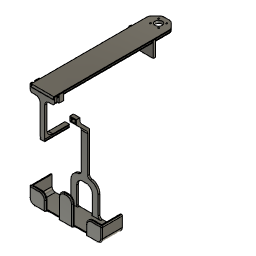
HeliumAntennaMount (Autodesk Fusion 360 design; units mm, degrees)
Autodesk Fusion 360 part; units mm, degrees
note: some values were not read from the file. Set by a fixed rule: which sketch regions a step uses.
sketch "Sketch1" plane through (0, 0, 0) normal (0, 0, 1) x (1, 0, 0)
  line L0 (0, -99.1) -> (0, 467.9) construction
  line L1 (-25, 0) -> (25, 0)
  line L2 (25, 0) -> (25, 275)
  line L3 (25, 275) -> (-25, 275)
  line L4 (-25, 275) -> (-25, 0)
  line L5 (-101.9, 257) -> (109.8, 257) construction
  circle A0 centre (0, 257) radius 8.12
  line L6 (-140.1, 0) -> (138.6, 0) construction
  dimension "d1" = 50
  dimension "d2" = 275
  dimension "d3" = 18
  dimension "d4" = 16.24
  constraint vertical L0
  constraint horizontal L1
  constraint vertical L2
  constraint horizontal L3
  constraint vertical L4
  constraint symmetric L0 L2 L4
  constraint perpendicular L2 L5
  constraint coincident L0 A0.centre
  constraint coincident L5 A0.centre
  constraint horizontal L6
  constraint collinear L1 L6
  measures "d1" distance of L1.start L1.end
  measures "d2" distance of L1.start L3.end
  measures "d3" distance of L3 L5
  measures "d4" diameter of A0
extrude "Extrude1" add sketch "Sketch1" along normal blind 6 makes body 1
sketch "Sketch2" plane through (0, 0, 0) normal (0, 0, -1) x (1, 0, 0)
  circle A0 centre (0, -257) radius 8.12
  line L0 (-25, 0) -> (-25, -275)
  line L1 (-25, -275) -> (25, -275)
  line L2 (25, -275) -> (25, 0)
  line L3 (25, 0) -> (-25, 0)
sketch "Sketch3" plane through (0, 0, 6) normal (0, 0, 1) x (-1, 0, 0)
  circle A0 centre (0, -257) radius 8.12
  line L0 (25, -275) -> (25, 0)
  line L1 (25, 0) -> (-25, 0)
  line L2 (-25, 0) -> (-25, -275)
  line L3 (-25, -275) -> (25, -275)
  line L4 (-9, -266) -> (9, -266) construction
  line L5 (9, -266) -> (9, -248) construction
  line L6 (9, -248) -> (-9, -248) construction
  line L7 (-9, -248) -> (-9, -266) construction
  line L8 (-9, -266) -> (9, -248) construction
  line L9 (9, -266) -> (-9, -248) construction
  circle A1 centre (9, -266) radius 1.625
  circle A2 centre (9, -248) radius 1.625
  circle A3 centre (-9, -248) radius 1.625
  circle A4 centre (-9, -266) radius 1.625
  point P0 (0, -257)
  dimension "d7" = 18
  dimension "d8" = 18
  dimension "d9" = 3.25
  dimension "d10" = 3.25
  dimension "d11" = 3.25
  dimension "d12" = 3.25
  constraint horizontal L4
  constraint perpendicular L4 L5
  constraint parallel L4 L6
  constraint parallel L5 L7
  constraint coincident L8 P0
  constraint coincident L9 P0
  constraint coincident P0 A0.centre
  constraint coincident L4.end L5.start
  constraint coincident L5.end L6.start
  constraint coincident L6.end L7.start
  constraint coincident L4.start L7.end
  measures "d7" distance of L5.end L6.end
  measures "d8" distance of L4.end L5.end
  measures "d9" diameter of A1
  measures "d10" diameter of A2
  measures "d11" diameter of A3
  measures "d12" diameter of A4
extrude "Extrude2" cut sketch "Sketch3" against normal up to surface (6 mm away) contours A1 | A2 | A3 | A4 bodies 1
chamfer "Chamfer1" distance 15 angle 45 1 edges at (-25, 275, 3) on bodies 1
chamfer "Chamfer2" distance 15 angle 45 1 edges at (25, 275, 3) on bodies 1
fillet "Fillet1" radius 10 4 edges at (10, 275, 3) (-10, 275, 3) (-25, 260, 3) (25, 260, 3) on bodies 1
sketch "Sketch6" plane through (0, 0, 0) normal (0, -1, 0) x (1, 0, 0)
  line L0 (-25, 0) -> (25, 0)
  line L1 (25, 0) -> (25, 6)
  line L2 (25, 6) -> (-25, 6)
  line L3 (-25, 6) -> (-25, 0)
  line L4 (-26.4781, 3) -> (26.4, 3) construction
  line L5 (-26.4, 4.5) -> (26.8, 4.5) construction
  line L6 (-26.4, 1.5) -> (26.8, 1.5) construction
  line L7 (-23.5, 6.3) -> (-23.5, 0.2) construction
  line L8 (-25, 1.5) -> (-23.5, 3)
  line L9 (-25, 4.5) -> (-23.5, 3)
  line L10 (0, 7.5) -> (0, -2.9) construction
  line L11 (25, 4.5) -> (23.5, 3)
  line L12 (25, 1.5) -> (23.5, 3)
  dimension "d28" = 1.5
  dimension "d29" = 1.5
  constraint perpendicular L1 L4
  constraint perpendicular L1 L5
  constraint symmetric L4 L5.start L6.start
  constraint symmetric L4 L5.end L6.end
  constraint perpendicular L6 L7
  constraint coincident L6 L8.start
  constraint coincident L3 L8.start
  constraint coincident L4 L8.end
  constraint coincident L7 L8.end
  constraint coincident L5 L9.start
  constraint coincident L3 L9.start
  constraint perpendicular L0 L10
  constraint symmetric L8.start L10 L12.start
  constraint symmetric L8.end L10 L11.end
  constraint symmetric L9.start L10 L11.start
  measures "d28" distance of L4 L5
  measures "d29" distance of L3 L7
extrude "Extrude6" cut sketch "Sketch6" against normal up to surface (275 mm away) contours L3 L8 L9 | L1 L11 L12 bodies 1
copy_body "Body->Comp1" bodies 1 removing the originals makes body 2 in component "Bodey"
sketch "Sketch1 (2)" plane through (0, 0, 0) normal (0, 1, 0) x (1, 0, 0) in component "Leg 1"
  line L0 (-25, -4.5) -> (-23.5, -3)
  line L1 (-23.5, -3) -> (-25, -1.5)
  line L2 (-25, -1.5) -> (-25, 0)
  line L3 (-25, 0) -> (25, 0)
  line L4 (25, 0) -> (25, -1.5)
  line L5 (25, -1.5) -> (23.5, -3)
  line L6 (23.5, -3) -> (25, -4.5)
  line L7 (25, -4.5) -> (25, -6)
  line L8 (-25, -6) -> (-25, -4.5)
  line L9 (-25.15, -6) -> (-25.15, -4.4379)
  line L10 (-25.15, -4.4379) -> (-23.7121, -3)
  line L11 (-23.7121, -3) -> (-25.15, -1.5621)
  line L12 (-25.15, -1.5621) -> (-25.15, 0.15)
  line L13 (-25.15, 0.15) -> (25.15, 0.15)
  line L14 (25.15, 0.15) -> (25.15, -1.5621)
  line L15 (25.15, -1.5621) -> (23.7121, -3)
  line L16 (23.7121, -3) -> (25.15, -4.4379)
  line L17 (25.15, -4.4379) -> (25.15, -6)
  line L18 (-25.15, -6) -> (-27.15, -6)
  line L19 (-27.15, -6) -> (-27.15, 10.15)
  line L20 (-27.15, 10.15) -> (0, 10.15)
  line L21 (0, 15.35) -> (0, 0.25) construction
  line L22 (25.15, -6) -> (27.15, -6)
  line L23 (27.15, -6) -> (27.15, 10.15)
  line L24 (27.15, 10.15) -> (0, 10.15)
  line L25 (-27.8377, 0.15) -> (28.2, 0.15) construction
  line L26 (-5, 10.15) -> (-5, 90.15)
  line L27 (5, 10.15) -> (5, 90.15)
  line L28 (-5, 90.15) -> (5, 90.15)
  dimension "d32" = -0.15
  dimension "d33" = 2
  dimension "d36" = 10
  dimension "d43" = 80
  dimension "d44" = 5
  constraint perpendicular L9 L18
  constraint perpendicular L18 L19
  constraint perpendicular L19 L20
  constraint perpendicular L3 L21
  constraint symmetric L9.start L21 L17.end
  constraint symmetric L18.end L21 L22.end
  constraint symmetric L19.end L21 L23.end
  constraint symmetric L20.end L21 L24.end
  constraint parallel L3 L25
  constraint coincident L20 L26.start
  constraint perpendicular L20 L26
  constraint symmetric L21 L26.start L27.start
  constraint symmetric L21 L26.end L27.end
  measures "d33" distance of L9.start L18.end
  measures "d36" distance of L20 L25
  measures "d43" distance of L26.start L26.end
  measures "d44" distance of L21 L26
extrude "Extrude5" add sketch "Sketch1 (2)" along normal blind 5 separate body makes body 3 in component "Leg 1"
extrude "Extrude3" add sketch "Sketch1 (2)" along normal blind 10 separate body contours L9 L10 L11 L12 L13 L14 L15 L16 L17 L18 L19 L20 L22 L23 L24 makes body 4 in component "Leg 1"
extrude "Extrude1'" add sketch "Sketch1 (2)" along normal blind 5 separate body contours L9 L10 L11 L12 L13 L14 L15 L16 L17 L18 L19 L20 L22 L23 L24 makes body 5 in component "Leg 1"
move_body "Move1" bodies 5 to x (1, 0, 0) y (0, 1, 0) z (0, 0, 1) at (0, 218.5, 0) in component "Leg 1"
sketch "Sketch2 (2)" plane through (0, 0, -10.15) normal (0, 0, -1) x (1, 0, 0) in component "Leg 1"
  line L0 (27.15, -218.5) -> (-27.15, -218.5)
  line L1 (-27.15, -218.5) -> (-27.15, -223.5)
  line L2 (-27.15, -223.5) -> (27.15, -223.5)
  line L3 (27.15, -223.5) -> (27.15, -218.5)
move_body "Move2" bodies 4 to x (1, 0, 0) y (0, 1, 0) z (0, 0, 1) at (0, 10, 0) in component "Leg 1"
extrude "Extrude4" add sketch "Sketch2 (2)" along normal blind 18.5 bodies 5 in component "Leg 1"
sketch "Sketch3 (2)" plane through (0, 5, 0) normal (0, 1, 0) x (-1, 0, 0) in component "Leg 1"
  line L0 (25.15, 6) -> (25.15, 4.4379)
  line L1 (25.15, 4.4379) -> (23.7121, 3)
  line L2 (23.7121, 3) -> (25.15, 1.5621)
  line L3 (25.15, 1.5621) -> (25.15, -0.15)
  line L4 (25.15, -0.15) -> (-25.15, -0.15)
  line L5 (-25.15, -0.15) -> (-25.15, 1.5621)
  line L6 (-25.15, 1.5621) -> (-23.7121, 3)
  line L7 (-23.7121, 3) -> (-25.15, 4.4379)
  line L8 (-25.15, 4.4379) -> (-25.15, 6)
  line L9 (-25.15, 6) -> (-27.15, 6)
  line L10 (-27.15, 6) -> (-27.15, -10.15)
  line L11 (-27.15, -10.15) -> (-5, -10.15)
  line L12 (-5, -10.15) -> (-5, -90.15)
  line L13 (-5, -90.15) -> (5, -90.15)
  line L14 (5, -90.15) -> (5, -10.15)
  line L15 (5, -10.15) -> (27.15, -10.15)
  line L16 (27.15, -10.15) -> (27.15, 6)
  line L17 (27.15, 6) -> (25.15, 6)
  line L18 (0, -57.1) -> (0, 9.3) construction
  line L19 (-5, -90.15) -> (5, -90.15)
  line L20 (5, -90.15) -> (5, -84.15)
  line L21 (5, -84.15) -> (-5, -84.15)
  line L22 (-5, -84.15) -> (-5, -90.15)
  dimension "d47" = 6
  constraint perpendicular L4 L18
  constraint horizontal L19
  constraint vertical L20
  constraint horizontal L21
  constraint vertical L22
  constraint coincident L12.end L13.start
  measures "d47" distance of L12.end L21.end
extrude "Extrude6'" add sketch "Sketch3 (2)" along normal blind 50 contours L12 L13 L14 L19 L20 L21 L22 bodies 3 in component "Leg 1"
sketch "Sketch4" plane through (0, 55, 0) normal (0, 1, 0) x (-1, 0, 0) in component "Leg 1"
  line L0 (-5, -84.15) -> (-5, -90.15)
  line L1 (-5, -90.15) -> (5, -90.15)
  line L2 (5, -90.15) -> (5, -84.15)
  line L3 (5, -84.15) -> (-5, -84.15)
  line L4 (-5, -87.15) -> (5, -87.15) construction
  line L5 (-5, -85.65) -> (5, -85.65) construction
  line L6 (-5, -88.65) -> (5, -88.65) construction
  line L7 (-3.5, -90.8) -> (-3.5, -84.15) construction
  line L8 (-3.5, -87.15) -> (-5, -88.65)
  line L9 (-3.5, -87.15) -> (-5, -85.65)
  line L10 (0, -91.3) -> (0, -83.7) construction
  line L11 (3.5, -87.15) -> (5, -85.65)
  line L12 (3.5, -87.15) -> (5, -88.65)
  dimension "d50" = 1.5
  dimension "d51" = 1.5
  constraint midpoint L0 L4.start
  constraint midpoint L2 L4.end
  constraint coincident L0 L5.start
  constraint coincident L2 L5.end
  constraint perpendicular L2 L5
  constraint symmetric L4 L5.start L6.start
  constraint symmetric L4 L5.end L6.end
  constraint coincident L3 L7.end
  constraint perpendicular L3 L7
  constraint coincident L4 L8.start
  constraint coincident L7 L8.start
  constraint perpendicular L3 L10
  constraint symmetric L5.start L10 L5.end
  constraint symmetric L6.start L10 L6.end
  constraint symmetric L8.start L10 L11.start
  measures "d50" distance of L4 L5
  measures "d51" distance of L0 L7
extrude "Extrude7" cut sketch "Sketch4" against normal up to surface (55 mm away) contours L0 L8 L9 | L2 L11 L12 bodies 3 in component "Leg 1"
fillet "Fillet1'" radius 13.25 1 edges at (0, 5, -84.15) on bodies 3 in component "Leg 1"
fillet "Fillet2" radius 10 1 edges at (-5, 2.5, -10.15) on bodies 3 in component "Leg 1"
fillet "Fillet3" radius 10 1 edges at (5, 2.5, -10.15) on bodies 3 in component "Leg 1"
fillet "Fillet4" radius 5 1 edges at (27.15, 2.5, -10.15) on bodies 3 in component "Leg 1"
fillet "Fillet5" radius 5 1 edges at (-27.15, 2.5, -10.15) on bodies 3 in component "Leg 1"
sketch "Sketch1 (3)" plane through (0, 55, 0) normal (0, 1, 0) x (-1, 0, 0) in component "Holster"
  line L0 (-3.5, -87.15) -> (-5, -88.65)
  line L1 (-5, -88.65) -> (-5, -90.15)
  line L2 (-5, -90.15) -> (5, -90.15)
  line L3 (5, -90.15) -> (5, -88.65)
  line L4 (5, -88.65) -> (3.5, -87.15)
  line L5 (3.5, -87.15) -> (5, -85.65)
  line L6 (5, -85.65) -> (5, -84.15)
  line L7 (5, -84.15) -> (-5, -84.15)
  line L8 (-5, -84.15) -> (-5, -85.65)
  line L9 (-5, -85.65) -> (-3.5, -87.15)
  line L10 (-5.15, -85.7121) -> (-3.7121, -87.15)
  line L11 (-3.7121, -87.15) -> (-5.15, -88.5879)
  line L12 (-5.15, -88.5879) -> (-5.15, -90.3)
  line L13 (-5.15, -90.3) -> (5.15, -90.3)
  line L14 (5.15, -90.3) -> (5.15, -88.5879)
  line L15 (5.15, -88.5879) -> (3.7121, -87.15)
  line L16 (3.7121, -87.15) -> (5.15, -85.7121)
  line L17 (5.15, -85.7121) -> (5.15, -84)
  line L18 (5.15, -84) -> (-5.15, -84)
  line L19 (-5.15, -84) -> (-5.15, -85.7121)
  line L20 (-7.15, -82) -> (7.15, -82)
  line L21 (7.15, -82) -> (7.15, -92.3)
  line L22 (7.15, -92.3) -> (-7.15, -92.3)
  line L23 (-7.15, -92.3) -> (-7.15, -82)
  dimension "d59" = 0.15
  dimension "d60" = 2
  dimension "d61" = 2
  dimension "d62" = 2
  dimension "d63" = 2
  constraint horizontal L20
  constraint vertical L21
  constraint horizontal L22
  constraint vertical L23
  measures "d60" distance of L18 L20
  measures "d61" distance of L13 L22
  measures "d62" distance of L12 L23
  measures "d63" distance of L14 L21
extrude "Extrude1''" add sketch "Sketch1 (3)" along normal blind 8 separate body contours L20 L21 L22 L23 makes body 6 in component "Holster"
ref_plane "WorkPlane1" through (7.15, 59, -87.15) normal (1, 0, 0) x (0, 0, -1)
sketch "Sketch7" plane through (7.15, 59, -87.15) normal (1, 0, 0) x (0, 1, 0)
  line L0 (-4, -5.15) -> (17.2132, -26.3632)
  line L1 (-4, -5.15) -> (26, -5.15) construction
  line L2 (17.2132, -26.3632) -> (25.2132, -26.3632)
  line L3 (25.2132, -26.3632) -> (4, -5.15)
  line L4 (4, -5.15) -> (-4, -5.15)
  point P0 (-4, -5.15)
  point P1 (4, -5.15)
  dimension "d67" = 30
  dimension "d68" = 45
  dimension "d69" = 8
  constraint horizontal L1
  constraint coincident P0 L0.start
  constraint horizontal L2
  constraint coincident P1 L3.end
  measures "d67" distance of P0 L0.end
  measures "d68" angle of L0 L1
  measures "d69" distance of L0.end L2.end
extrude "Extrude2'" add sketch "Sketch7" against normal blind 14.3 bodies 6 in component "Holster"
sketch "Sketch8" plane through (-7.15, 0, 0) normal (-1, 0, 0) x (0, -1, 0)
  line L0 (-55, -92.3) -> (-55, -82)
  line L1 (-55, -82) -> (-63, -82)
  line L2 (-63, -82) -> (-63, -92.3)
  line L3 (-63, -92.3) -> (-84.2132, -113.5132)
  line L4 (-84.2132, -113.5132) -> (-76.2132, -113.5132)
  line L5 (-76.2132, -113.5132) -> (-55, -92.3)
  line L6 (-84.2132, -113.5132) -> (-84.2132, -273.5132)
  line L7 (-84.2132, -273.5132) -> (-80.2132, -273.5132)
  line L8 (-80.2132, -273.5132) -> (-80.2132, -113.5132)
  dimension "d73" = 160
  dimension "d74" = 4
  constraint coincident L3.end L4.start
  constraint perpendicular L4 L6
  constraint perpendicular L6 L7
  constraint midpoint L4 L8.end
  measures "d73" distance of L3.end L6.end
  measures "d74" distance of L6.end L7.end
extrude "Extrude3'" add sketch "Sketch8" against normal up to surface (14.3 mm away) contours L4 L6 L7 L8 bodies 6 in component "Holster"
fillet "Fillet1''" radius 13 1 edges at (0, 63, -92.3) on bodies 6 in component "Holster"
fillet "Fillet2'" radius 9.5 1 edges at (0, 80.2132, -113.5132) on bodies 6 in component "Holster"
sketch "Sketch18" plane through (0, 0, -273.5132) normal (0, 0, -1) x (1, 0, 0)
  line L0 (7.15, -84.2132) -> (7.15, -80.2132)
  line L1 (7.15, -80.2132) -> (-7.15, -80.2132)
  line L2 (-7.15, -80.2132) -> (-7.15, -84.2132)
  line L3 (-7.15, -84.2132) -> (7.15, -84.2132)
  line L4 (0, -80.2132) -> (0, -85.7)
  line L5 (-76, -42.2132) -> (76, -42.2132)
  line L6 (76, -42.2132) -> (76, -80.2132)
  line L7 (76, -80.2132) -> (-76, -80.2132)
  line L8 (-76, -80.2132) -> (-76, -42.2132)
  dimension "d134" = 152
  dimension "d135" = 38
  constraint midpoint L1 L4.start
  constraint perpendicular L3 L4
  constraint horizontal L5
  constraint vertical L6
  constraint horizontal L7
  constraint vertical L8
  constraint midpoint L4.start L7
  measures "d134" distance of L5.start L5.end
  measures "d135" distance of L5.start L7.end
extrude "Extrude7'" add sketch "Sketch18" along normal blind 4 separate body contours L1 L5 L6 L7 L8 makes body 7
sketch "Sketch19" plane through (0, 80.2132, 0) normal (0, 1, 0) x (-1, 0, 0)
  line L0 (76, -273.5132) -> (-76, -273.5132)
  line L1 (-76, -273.5132) -> (-76, -277.5132)
  line L2 (-76, -277.5132) -> (76, -277.5132)
  line L3 (76, -277.5132) -> (76, -273.5132)
extrude "Extrude8" add sketch "Sketch19" along normal up to surface (4 mm away) bodies 7
sketch "Sketch20" plane through (-76, 0, 0) normal (-1, 0, 0) x (0, -1, 0)
  line L0 (-42.2132, -273.5132) -> (-84.2132, -273.5132)
  line L1 (-84.2132, -273.5132) -> (-84.2132, -277.5132)
  line L2 (-84.2132, -277.5132) -> (-42.2132, -277.5132)
  line L3 (-42.2132, -277.5132) -> (-42.2132, -273.5132)
  line L4 (-42.2132, -277.5132) -> (-103.2132, -277.5132)
  line L5 (-103.2132, -277.5132) -> (-103.2132, -242.5132)
  line L6 (-103.2132, -242.5132) -> (-42.2132, -242.5132)
  line L7 (-42.2132, -242.5132) -> (-42.2132, -277.5132)
  dimension "d140" = 35
  constraint horizontal L4
  constraint vertical L5
  constraint horizontal L6
  constraint vertical L7
  constraint coincident L2.end L3.start
  measures "d140" distance of L2.end L6.end
extrude "Extrude9" add sketch "Sketch20" along normal blind 4 separate body contours L0 L1 L4 L5 L6 L7 makes body 8
sketch "Sketch21" plane through (0, 0, -273.5132) normal (0, 0, -1) x (1, 0, 0)
  line L0 (-76, -84.2132) -> (-76, -42.2132)
  line L1 (-76, -42.2132) -> (-80, -42.2132)
  line L2 (-80, -42.2132) -> (-80, -84.2132)
  line L3 (-80, -84.2132) -> (-76, -84.2132)
extrude "Extrude10" add sketch "Sketch21" along normal up to surface (4 mm away) bodies 7 8
ref_plane "WorkPlane3" through (76, 72.7132, -260.0132) normal (1, 0, 0) x (0, 1, 0)
sketch "Sketch22" plane through (76, 53.7132, -258.0132) normal (1, 0, 0) x (0, 1, 0)
  line L0 (49.5, -19.5) -> (-11.5, -19.5)
  line L1 (-11.5, -19.5) -> (-11.5, 15.5)
  line L2 (-11.5, 15.5) -> (49.5, 15.5)
  line L3 (49.5, 15.5) -> (49.5, -19.5)
extrude "Extrude11" add sketch "Sketch22" along normal blind 4 bodies 7
sketch "Sketch23" plane through (0, 42.2132, 0) normal (0, -1, 0) x (1, 0, 0)
  line L0 (-80, -242.5132) -> (-80, -277.5132)
  line L1 (-80, -277.5132) -> (80, -277.5132)
  line L2 (80, -277.5132) -> (80, -242.5132)
  line L3 (80, -242.5132) -> (76, -242.5132)
  line L4 (76, -242.5132) -> (76, -273.5132)
  line L5 (76, -273.5132) -> (-76, -273.5132)
  line L6 (-76, -273.5132) -> (-76, -242.5132)
  line L7 (-76, -242.5132) -> (-80, -242.5132)
  line L8 (-80, -242.5132) -> (-45, -242.5132)
  line L9 (-45, -242.5132) -> (-45, -277.5132)
  line L10 (-45, -277.5132) -> (-80, -277.5132)
  line L11 (-80, -277.5132) -> (-80, -242.5132)
  line L12 (80, -242.5132) -> (45, -242.5132)
  line L13 (45, -242.5132) -> (45, -277.5132)
  line L14 (45, -277.5132) -> (80, -277.5132)
  line L15 (80, -277.5132) -> (80, -242.5132)
  dimension "d148" = 35
  dimension "d149" = 35
  constraint horizontal L8
  constraint vertical L9
  constraint horizontal L10
  constraint vertical L11
  constraint coincident L1 L9.end
  constraint coincident L0.start L7.end
  constraint horizontal L12
  constraint vertical L13
  constraint horizontal L14
  constraint vertical L15
  constraint coincident L1 L13.end
  constraint coincident L2.end L3.start
  measures "d148" distance of L0.start L8.end
  measures "d149" distance of L2.end L12.end
extrude "Extrude12" add sketch "Sketch23" along normal blind 4 contours L0 L1 L5 L6 L7 L8 L9 L10 L11 | L5 L6 L8 L9 | L1 L2 L3 L4 L5 L12 L13 L14 L15 | L4 L5 L12 L13 bodies 7
sketch "Sketch24" plane through (0, 42.2132, 0) normal (0, -1, 0) x (1, 0, 0)
  line L0 (-45, -273.5132) -> (-45, -277.5132)
  line L1 (-45, -277.5132) -> (45, -277.5132)
  line L2 (45, -277.5132) -> (45, -273.5132)
  line L3 (45, -273.5132) -> (-45, -273.5132)
  line L4 (7.15, -273.5132) -> (7.15, -121.2592)
  line L5 (-26.7, -248.5132) -> (32.5, -248.5132) construction
  line L6 (-15.1892, -277.5132) -> (15.1892, -277.5132)
  line L7 (15.1892, -277.5132) -> (15.1892, -219.5132)
  line L8 (15.1892, -219.5132) -> (-15.1892, -219.5132)
  line L9 (-15.1892, -219.5132) -> (-15.1892, -277.5132)
  line L10 (-15.1892, -277.5132) -> (15.1892, -219.5132) construction
  line L11 (15.1892, -277.5132) -> (-15.1892, -219.5132) construction
  point P0 (0, -248.5132)
  dimension "d152" = 25
  constraint perpendicular L4 L5
  constraint horizontal L6
  constraint perpendicular L6 L7
  constraint parallel L6 L8
  constraint parallel L7 L9
  constraint coincident L1 L6.start
  constraint coincident L10 P0
  constraint coincident L11 P0
  constraint coincident L5 P0
  measures "d152" distance of L3 L5.start
extrude "Extrude13" add sketch "Sketch24" along normal blind 4 contours L3 L4 L8 L9 | L1 L3 L6 L7 L9 | L3 L4 L7 L8 bodies 7
fillet "Fillet2''" radius 10.9 2 edges at (80, 70.7132, -277.5132) (-80, 70.7132, -277.5132) on bodies 7
fillet "Fillet3'" radius 7.45 2 edges at (-76, 63.2132, -273.5132) (76, 63.2132, -273.5132) on bodies 7
sketch "Sketch25" plane through (0, 0, -273.5132) normal (0, 0, -1) x (1, 0, 0)
  line L0 (7.15, -84.2132) -> (7.15, -80.2132)
  line L1 (7.15, -80.2132) -> (-7.15, -80.2132)
  line L2 (-7.15, -80.2132) -> (-7.15, -84.2132)
  line L3 (-7.15, -84.2132) -> (7.15, -84.2132)
extrude "Extrude15" add sketch "Sketch25" along normal up to surface (4 mm away) bodies 6 in component "Holster"
copy_body "CutPasteBodies1" bodies 7 removing the originals makes body 9 in component "Holster"
combine "Combine1" operation add target body 6 tool bodies 9 in component "Holster"
fillet "Fillet15" radius 5.75 2 edges at (7.15, 82.2132, -273.5132) (-7.15, 82.2132, -273.5132) on bodies 6 in component "Holster"
fillet "Fillet16" radius 12.75 4 edges at (-45, 40.2132, -242.5132) (45, 40.2132, -242.5132) (-15.1892, 40.2132, -219.5132) (15.1892, 40.2132, -219.5132) on bodies 6 in component "Holster"
fillet "Fillet17" radius 2 13 edges at (-45, 38.2132, -266.3882) (-48.7344, 38.2132, -246.2476) (-68.875, 38.2132, -242.5132) (-80, 70.7132, -242.5132) (15.1892, 38.2132, -254.8882) (11.4548, 38.2132, -223.2476) (0, 38.2132, -219.5132) (-11.4548, 38.2132, -223.2476) (-15.1892, 38.2132, -254.8882) (68.875, 38.2132, -242.5132) (48.7344, 38.2132, -246.2476) (45, 38.2132, -266.3882) (80, 70.7132, -242.5132) on bodies 6 in component "Holster"
fillet "Fillet18" radius 3.05 4 edges at (-45, 42.2132, -275.5132) (15.1892, 42.2132, -275.5132) (45, 42.2132, -275.5132) (-15.1892, 42.2132, -275.5132) on bodies 6 in component "Holster"
fillet "Fillet19" radius 2 1 edges at (0, 80.2132, -273.5132) on bodies 6 in component "Holster"
ref_plane "WorkPlane4" through (0, 84.2132, -195.5132) normal (0, 1, 0) x (0, 0, 1)
sketch "Sketch26" plane through (0, 84.2132, -195.5132) normal (0, 1, 0) x (1, 0, 0)
  arc A0 (2.4392, 24) -> (15.1892, 36.75) centre (2.4392, 36.75) ccw
  line L0 (15.1892, 36.75) -> (15.1892, 78)
  line L1 (15.1892, 78) -> (-15.1892, 78)
  line L2 (-15.1892, 78) -> (-15.1892, 36.75)
  arc A1 (-15.1892, 36.75) -> (-2.4392, 24) centre (-2.4392, 36.75) ccw
  line L3 (-2.4392, 24) -> (2.4392, 24)
  line L4 (12.9, 78) -> (-12.9, 78)
  line L5 (-12.9, 78) -> (-68.55, 78)
  line L6 (-68.55, 78) -> (-45, 78)
  line L7 (-45.0437, 78) -> (-45, 78)
  line L8 (-42.0604, 78) -> (-45.0437, 78)
  line L9 (-42.0604, 78) -> (-18.1289, 78)
  line L10 (-18.1289, 78) -> (-15.1455, 78)
  line L11 (-15.1892, 78) -> (-15.1455, 78)
  line L12 (-15.1892, 78) -> (15.1892, 78)
  line L13 (15.1455, 78) -> (15.1892, 78)
  line L14 (18.1289, 78) -> (15.1455, 78)
  line L15 (18.1289, 78) -> (42.0604, 78)
  line L16 (42.0604, 78) -> (45.0437, 78)
  line L17 (45, 78) -> (45.0437, 78)
  line L18 (45, 78) -> (68.55, 78)
  line L19 (68.55, 78) -> (12.9, 78)
  line L20 (30, 78) -> (-30, 78)
  line L21 (-30, 78) -> (-30, 11.9)
  line L22 (-30, 11.9) -> (30, 11.9)
  line L23 (30, 11.9) -> (30, 78)
  line L24 (0, 111.7) -> (0, 6.8) construction
  line L25 (-2.4392, 21.7283) -> (2.4392, 21.7283)
  arc A2 (2.4392, 21.7283) -> (17.4609, 36.75) centre (2.4392, 36.75) ccw
  line L26 (17.4609, 36.75) -> (17.4609, 80.2717)
  line L27 (17.4609, 80.2717) -> (-17.4609, 80.2717)
  line L28 (-17.4609, 80.2717) -> (-17.4609, 36.75)
  arc A3 (-17.4609, 36.75) -> (-2.4392, 21.7283) centre (-2.4392, 36.75) ccw
  dimension "d166" = 60
  dimension "d167" = 2.2717
  constraint horizontal L20
  constraint vertical L21
  constraint horizontal L22
  constraint vertical L23
  constraint coincident L15 L20.start
  constraint perpendicular L22 L24
  constraint symmetric L21 L23 L24
  measures "d166" distance of L20.start L20.end
extrude "Extrude16" add sketch "Sketch26" against normal blind 4 contours L5 L9 L10 L14 L15 L19 L20 L21 L22 L23 L25 A2 L26 L28 A3 bodies 6 in component "Holster"
sketch "Sketch27" plane through (0, 84.2132, 0) normal (0, 1, 0) x (-1, 0, 0)
  line L0 (-30, -273.5132) -> (-68.55, -273.5132)
  arc A0 (-76, -266.0632) -> (-68.55, -273.5132) centre (-68.55, -266.0632) ccw
  line L1 (-76, -266.0632) -> (-76, -275.0512)
  arc A1 (-76, -275.0512) -> (-69.1, -277.5132) centre (-69.1, -266.6132) ccw
  line L2 (-69.1, -277.5132) -> (69.1, -277.5132)
  arc A2 (69.1, -277.5132) -> (76, -275.0512) centre (69.1, -266.6132) ccw
  line L3 (76, -275.0512) -> (76, -266.0632)
  arc A3 (68.55, -273.5132) -> (76, -266.0632) centre (68.55, -266.0632) ccw
  line L4 (68.55, -273.5132) -> (30, -273.5132)
  line L5 (30, -273.5132) -> (30, -207.4132)
  line L6 (30, -207.4132) -> (7.15, -207.4132)
  line L7 (7.15, -207.4132) -> (7.15, -113.5132)
  line L8 (7.15, -113.5132) -> (-7.15, -113.5132)
  line L9 (-7.15, -113.5132) -> (-7.15, -207.4132)
  line L10 (-7.15, -207.4132) -> (-30, -207.4132)
  line L11 (-30, -207.4132) -> (-30, -273.5132)
  line L12 (-17.4609, -273.5132) -> (-17.4609, -232.2632)
  arc A4 (-7.15, -217.9993) -> (-17.4609, -232.2632) centre (-2.4392, -232.2632) ccw
  line L13 (-7.15, -217.9993) -> (-7.15, -267.7632)
  arc A5 (-12.9, -273.5132) -> (-7.15, -267.7632) centre (-12.9, -267.7632) ccw
  line L14 (-12.9, -273.5132) -> (-17.4609, -273.5132)
  arc A6 (17.4609, -232.2632) -> (7.15, -217.9993) centre (2.4392, -232.2632) ccw
  line L15 (17.4609, -232.2632) -> (17.4609, -273.5132)
  line L16 (17.4609, -273.5132) -> (12.9, -273.5132)
  arc A7 (7.15, -267.7632) -> (12.9, -273.5132) centre (12.9, -267.7632) ccw
  line L17 (7.15, -267.7632) -> (7.15, -217.9993)
  arc A8 (-2.4392, -219.5132) -> (-15.1892, -232.2632) centre (-2.4392, -232.2632) ccw
  line L18 (-15.1892, -232.2632) -> (-15.1892, -273.5132)
  line L19 (-15.1892, -273.5132) -> (15.1892, -273.5132)
  line L20 (15.1892, -273.5132) -> (15.1892, -232.2632)
  arc A9 (15.1892, -232.2632) -> (2.4392, -219.5132) centre (2.4392, -232.2632) ccw
  line L21 (2.4392, -219.5132) -> (-2.4392, -219.5132)
extrude "Extrude17" cut sketch "Sketch27" against normal blind 14.5 contours L13 A5 A7 L17 A8 L19 A9 L21 bodies 6 in component "Holster"
sketch "Sketch28" plane through (0, 84.2132, 0) normal (0, 1, 0) x (-1, 0, 0)
  arc A0 (-2.4392, -219.5132) -> (-7.15, -220.4154) centre (-2.4392, -232.2632) ccw
  line L0 (-2.4392, -219.5132) -> (2.4392, -219.5132)
  arc A1 (7.15, -220.4154) -> (2.4392, -219.5132) centre (2.4392, -232.2632) ccw
  line L1 (7.15, -220.4154) -> (7.15, -217.9993)
  arc A2 (17.4609, -232.2632) -> (7.15, -217.9993) centre (2.4392, -232.2632) ccw
  line L2 (17.4609, -232.2632) -> (17.4609, -273.5132)
  line L3 (17.4609, -273.5132) -> (-17.4609, -273.5132)
  line L4 (-17.4609, -273.5132) -> (-17.4609, -232.2632)
  arc A3 (-7.15, -217.9993) -> (-17.4609, -232.2632) centre (-2.4392, -232.2632) ccw
  line L5 (-7.15, -217.9993) -> (-7.15, -220.4154)
  line L6 (-30, -273.5132) -> (-68.55, -273.5132)
  arc A4 (-76, -266.0632) -> (-68.55, -273.5132) centre (-68.55, -266.0632) ccw
  line L7 (-76, -266.0632) -> (-76, -275.0512)
  arc A5 (-76, -275.0512) -> (-69.1, -277.5132) centre (-69.1, -266.6132) ccw
  line L8 (-69.1, -277.5132) -> (69.1, -277.5132)
  arc A6 (69.1, -277.5132) -> (76, -275.0512) centre (69.1, -266.6132) ccw
  line L9 (76, -275.0512) -> (76, -266.0632)
  arc A7 (68.55, -273.5132) -> (76, -266.0632) centre (68.55, -266.0632) ccw
  line L10 (68.55, -273.5132) -> (30, -273.5132)
  line L11 (30, -273.5132) -> (30, -207.4132)
  line L12 (30, -207.4132) -> (7.15, -207.4132)
  line L13 (7.15, -207.4132) -> (7.15, -113.5132)
  line L14 (7.15, -113.5132) -> (-7.15, -113.5132)
  line L15 (-7.15, -113.5132) -> (-7.15, -207.4132)
  line L16 (-7.15, -207.4132) -> (-30, -207.4132)
  line L17 (-30, -207.4132) -> (-30, -273.5132)
  line L18 (-7.15, -217.9993) -> (7.15, -217.9993)
  constraint coincident A3.start L5.start
  constraint coincident L1.end A2.end
extrude "Extrude18" cut sketch "Sketch28" against normal blind 5.3 contours A0 L0 A1 L1 L5 L18 bodies 6 in component "Holster"
fillet "Fillet20" radius 19.4 2 edges at (-30, 82.2132, -207.4132) (30, 82.2132, -207.4132) on bodies 6 in component "Holster"
fillet "Fillet21" radius 6.3 2 edges at (7.15, 82.2132, -207.4132) (-7.15, 82.2132, -207.4132) on bodies 6 in component "Holster"
fillet "Fillet22" radius 2 19 edges at (-79.4142, 38.799, -243.099) (-80, 38.2132, -255.5632) (-76.8075, 38.2132, -274.3207) (-58.05, 38.2132, -277.5132) (-45.7414, 38.6589, -277.5132) (-43.9798, 41.5335, -277.5132) (-30.0946, 42.2132, -277.5132) (-16.2094, 41.5335, -277.5132) (-14.4479, 38.6589, -277.5132) (0, 38.2132, -277.5132) (14.4479, 38.6589, -277.5132) (16.2094, 41.5335, -277.5132) (30.0946, 42.2132, -277.5132) (43.9798, 41.5335, -277.5132) (45.7414, 38.6589, -277.5132) (58.05, 38.2132, -277.5132) (76.8075, 38.2132, -274.3207) (80, 38.2132, -255.5632) (79.4142, 38.799, -243.099) on bodies 6 in component "Holster"
fillet "Fillet23" radius 2 2 edges at (17.4609, 82.2132, -273.5132) (-17.4609, 82.2132, -273.5132) on bodies 6 in component "Holster"
fillet "Fillet24" radius 6 2 edges at (-30, 82.2132, -273.5132) (30, 82.2132, -273.5132) on bodies 6 in component "Holster"
sketch "Sketch29" plane through (0, 38.2132, 0) normal (0, -1, 0) x (1, 0, 0)
  line L0 (-1.2143, -278.7905) -> (25.1641, -278.7905)
  line L1 (25.1641, -278.7905) -> (25.1641, -235.5405)
  arc A0 (25.1641, -235.5405) -> (14.4141, -224.7905) centre (14.4141, -235.5405) ccw
  line L2 (14.4141, -224.7905) -> (9.5357, -224.7905)
  arc A1 (9.5357, -224.7905) -> (-1.2143, -235.5405) centre (9.5357, -235.5405) ccw
  line L3 (-1.2143, -235.5405) -> (-1.2143, -278.7905)
ref_plane "WorkPlane5" through (11.9749, 61.2132, -280.7905) normal (0, 0, -1) x (-1, 0, 0)
sketch "Sketch30" plane through (11.9749, 52.7132, -280.7905) normal (0, 0, -1) x (1, 0, 0)
sketch "Sketch31" plane through (0, -12.6189, 0) normal (0, 1, 0) x (-1, 0, 0)
  arc A0 (-167.915, -207.1178) -> (-185.1636, -226.3981) centre (-165.7636, -226.3981) ccw
  line L0 (-185.1636, -226.3981) -> (-185.1636, -267.0981)
  arc A1 (-191.1636, -273.0981) -> (-185.1636, -267.0981) centre (-191.1636, -267.0981) ccw
  line L1 (-191.1636, -273.0981) -> (-223.7136, -273.0981)
  arc A2 (-231.1636, -265.6481) -> (-223.7136, -273.0981) centre (-223.7136, -265.6481) ccw
  line L2 (-231.1636, -265.6481) -> (-231.1636, -274.6362)
  arc A3 (-231.1636, -274.6362) -> (-224.2636, -277.0981) centre (-224.2636, -266.1981) ccw
  line L3 (-224.2636, -277.0981) -> (-86.0636, -277.0981)
  arc A4 (-86.0636, -277.0981) -> (-79.1636, -274.6362) centre (-86.0636, -266.1981) ccw
  line L4 (-79.1636, -274.6362) -> (-79.1636, -265.6481)
  arc A5 (-86.6136, -273.0981) -> (-79.1636, -265.6481) centre (-86.6136, -265.6481) ccw
  line L5 (-86.6136, -273.0981) -> (-119.1636, -273.0981)
  arc A6 (-125.1636, -267.0981) -> (-119.1636, -273.0981) centre (-119.1636, -267.0981) ccw
  line L6 (-125.1636, -267.0981) -> (-125.1636, -226.3981)
  arc A7 (-125.1636, -226.3981) -> (-142.4123, -207.1178) centre (-144.5636, -226.3981) ccw
  arc A8 (-148.0136, -200.8567) -> (-142.4123, -207.1178) centre (-141.7136, -200.8567) ccw
  line L7 (-148.0136, -200.8567) -> (-148.0136, -113.0981)
  line L8 (-148.0136, -113.0981) -> (-162.3136, -113.0981)
  line L9 (-162.3136, -113.0981) -> (-162.3136, -200.8567)
  arc A9 (-167.915, -207.1178) -> (-162.3136, -200.8567) centre (-168.6136, -200.8567) ccw
  line L10 (-162.3136, -217.5842) -> (-148.0136, -217.5842)
  arc A10 (-137.7027, -231.8481) -> (-148.0136, -217.5842) centre (-152.7244, -231.8481) ccw
  line L11 (-137.7027, -231.8481) -> (-137.7027, -271.0981)
  arc A11 (-139.7027, -273.0981) -> (-137.7027, -271.0981) centre (-139.7027, -271.0981) ccw
  line L12 (-139.7027, -273.0981) -> (-170.6245, -273.0981)
  arc A12 (-172.6245, -271.0981) -> (-170.6245, -273.0981) centre (-170.6245, -271.0981) ccw
  line L13 (-172.6245, -271.0981) -> (-172.6245, -231.8481)
  arc A13 (-162.3136, -217.5842) -> (-172.6245, -231.8481) centre (-157.6028, -231.8481) ccw
  line L14 (-250.1931, -277.0981) -> (-71, -277.0981)
  line L15 (-71, -277.0981) -> (-71, -229.9)
  line L16 (-71, -229.9) -> (-250.1931, -229.9)
  line L17 (-250.1931, -229.9) -> (-250.1931, -277.0981)
  constraint horizontal L14
  constraint vertical L15
  constraint horizontal L16
  constraint vertical L17
extrude "Extrude19" cut sketch "Sketch31" along normal blind 24.6 contours L0 A1 L1 A2 L2 A3 L3 A4 L4 A5 L5 A6 L6 A10 L11 A11 L12 A12 L13 A13 L14 L16 | L0 A1 L1 A2 L2 A3 L14 L16 L17 | A4 L4 A5 L5 A6 L6 L14 L15 L16 sketch seen with x (1, 0, 0) y (0, 1, 0) z (0, 0, 1) at (-155.1636, 96.8321, -0.4151) bodies 6 in component "Holster"
component "Bodey" placed x (1, 0, 0) y (0, 1, 0) z (0, 0, 1) at (0, 0, 0)
component "Leg 1" placed x (1, 0, 0) y (0, 1, 0) z (0, 0, 1) at (0, 0, 0)
component "Hanger" placed x (1, 0, 0) y (0, 1, 0) z (0, 0, 1) at (0, 0, 0)
component "Holster" placed x (1, 0, 0) y (0, 1, 0) z (0, 0, 1) at (155.1636, -96.8321, 0.4151)
